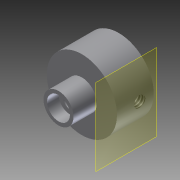
# Autodesk Inventor part: bottom_cap
Saved by Autodesk Inventor 2011 SP2 (Build 150309200, 309)
## iProperties
Created: 2013-09-16
Part Number: bottom_cap
Document SubType Name: Modeling
Designer: sungwook
Density: 1 g/cm^3
Author: sungwook
Autodesk Inventor part; units mm, degrees
ref_plane "XZ Plane" through (0, 0, 0) normal (0, 1, 0) x (-1, 0, 0)
ref_plane "XY Plane" through (0, 0, 0) normal (0, 0, 1) x (1, 0, 0)
sketch "Sketch1" plane through (0, 0, 0) normal (0, 0, 1) x (1, 0, 0)
  circle A0 centre (0, 0) radius 3.81
  dimension "d0" = 7.62
  constraints: 1 centre point, 1 coincident
  measures "d0" diameter of A0
extrude "Extrusion1" add sketch "Sketch1" along normal blind 4
sketch "Sketch2" plane through (0, 0, 4) normal (0, 0, 1) x (1, 0, 0)
  circle A0 centre (0, 0) radius 3.81 projected
  circle A1 centre (0, 0) radius 1.6256
  dimension "d3" = 3.2512
  constraints: 1 centre point, 1 coincident
  measures "d3" diameter of A1
extrude "Extrusion2" add sketch "Sketch2" along normal blind 2.54 contours A1
sketch "Sketch3" plane through (0, 0, 6.54) normal (0, 0, 1) x (1, 0, 0)
  circle A0 centre (0, 0) radius 1.6256 projected
hole "Hole1" at (0, 0, 6.54) direction (0, 0, -1) diameter 1.524 end through all
sketch "Sketch4" plane through (0, 0, 0) normal (0, 0, -1) x (-1, 0, 0)
  circle A0 centre (0, 0) radius 0.762 projected
  circle A1 centre (0, 0) radius 3.81 projected
  circle A2 centre (0, 0) radius 2.159
  dimension "d15" = 4.318
  constraints: 1 centre point, 1 coincident
  measures "d15" diameter of A2
extrude "Extrusion3" cut sketch "Sketch4" against normal blind 3 contours A2
ref_plane "Work Plane1" through (3.81, 0, 0) normal (1, 0, 0) x (0, 1, 0)
sketch "Sketch5" plane through (3.81, 0, 0) normal (1, 0, 0) x (0, 1, 0)
  line L0 (-3.81, 4) -> (3.81, 4) projected
  line L1 (-3.81, 0) -> (3.81, 0) projected
  line L2 (0, -1.2) -> (0, 7.2) projected
  line L3 (-2.159, 3) -> (2.159, 3) projected
  point P0 (0, 0)
  point P1 (0, 1.524)
  dimension "d16" = 3
  dimension "d17" = 1.524
  constraints: 1 point on line
  measures "d16" distance between parallel lines of L1 L3
  measures "d17" distance from line of L1 point (0, 1.524)
hole "Hole2" at (3.81, 0, 1.524) direction (-1, 0, 0) diameter 1.1938 end up to face face through (0, 0, 0) facing (0, 0, 1) round with radius 2.159 far side yes
sketch "Sketch6" plane through (0, 0, 6.54) normal (0, 0, 1) x (1, 0, 0)
  circle A0 centre (0, 0) radius 0.762 projected
  circle A1 centre (0, 0) radius 1.6256 projected
  circle A2 centre (0, 0) radius 1.2446
  dimension "d25" = 2.4892
  constraints: 1 centre point, 1 coincident
  measures "d25" diameter of A2
extrude "Extrusion4" cut sketch "Sketch6" against normal blind 1.27 contours A2
body "Solid1"
